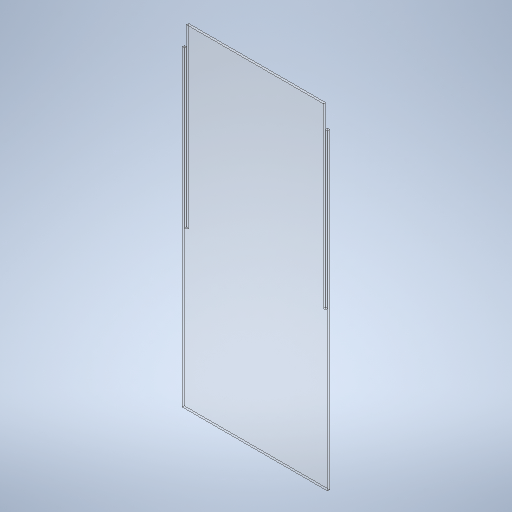
# Autodesk Inventor part: Finishing Sheets .4 ( Front )  Acrylic
Saved by Autodesk Inventor 2025.4 (Build 294407000, 407)
## iProperties
Created: 2026-04-04
Part Number: Finishing Sheets .4 ( Front )  Acrylic
Material: PMMA Plastic
Document SubType Name: Sheet Metal
Designer: lenovo
Density: 1.188 g/cm^3
Sheet Metal Rule: Default_mm
Appearance: Polycarbonate - Clear
Author: lenovo
Autodesk Inventor part; units mm, degrees
ref_plane "YZ Plane" through (0, 0, 0) normal (1, 0, 0) x (0, 1, 0)
ref_plane "XZ Plane" through (0, 0, 0) normal (0, 1, 0) x (-1, 0, 0)
ref_plane "XY Plane" through (0, 0, 0) normal (0, 0, 1) x (1, 0, 0)
sketch "Sketch1" plane through (0, 0, 0) normal (0, 0, 1) x (1, 0, 0)
  line L0 (-102.5, -220) -> (102.5, -220)
  line L1 (102.5, -220) -> (102.5, 220)
  line L2 (102.5, 220) -> (-102.5, 220)
  line L3 (-102.5, 220) -> (-102.5, -220)
  line L4 (-102.5, -220) -> (102.5, 220) construction
  line L5 (102.5, -220) -> (-102.5, 220) construction
  line L6 (-96.5, 220) -> (-99.5, 220)
  line L7 (-99.5, 220) -> (-99.5, 0)
  line L8 (-99.5, 0) -> (-96.5, 0)
  line L9 (-96.5, 0) -> (-96.5, 220)
  line L10 (0, 220) -> (0, 0)
  line L11 (99.5, 220) -> (99.5, 0)
  line L12 (99.5, 0) -> (96.5, 0)
  line L13 (96.5, 0) -> (96.5, 220)
  dimension "d0" = 205
  dimension "d1" = 440
  dimension "d2" = 3
  dimension "d3" = 3
  dimension "d4" = 220
  measures "d0" distance of L1.end L2.end
  measures "d1" distance of L0.end L1.end
  measures "d2" distance between parallel lines of L7 L9
  measures "d3" distance between parallel lines of L3 L7
  measures "d4" distance of L8.end L6.start
sketch "Sketch2" plane through (0, 0, 3) normal (0, 0, 1) x (1, 0, 0)
  line L0 (-96.5, 250) -> (96.5, 250)
  line L1 (96.5, 250) -> (96.5, 220)
  line L2 (96.5, 220) -> (-96.5, 220)
  line L3 (-96.5, 220) -> (-96.5, 250)
  line L4 (-96.5, 250) -> (96.5, 220) construction
  line L5 (96.5, 250) -> (-96.5, 220) construction
  line L6 (-96.5, 220) -> (96.5, 220)
  point P0 (0, 0)
  point P1 (0, 235)
  point P2 (0, 220)
  dimension "d6" = 30
  measures "d6" distance of L0.end L1.end
extrude "Plate1" add sketch "Sketch1" along normal blind 3 contours L3 L2 L7 L8 L9 L13 L12 L11 L1 L0
sheet face with bend "Face2" sketch "Sketch2" thickness 3 toward (0, 0, -1) bend radius 3
bend "Bend1"
equation "\"d5\" = Thickness"
equation "\"d7\" = BendRadius"
equation "\"d8\" = BendReliefWidth"
equation "\"d10\" = MinimumRemnant"
equation "\"d9\" = BendReliefDepth"
equation "\"d11\" = TransitionRadius"
equation "\"BendRadius\" = Thickness"
equation "\"BendReliefWidth\" = Thickness"
equation "\"BendReliefDepth\" = 0.5 * Thickness"
equation "\"CornerReliefSize\" = 4 * Thickness"
equation "\"MinimumRemnant\" = 2 * Thickness"
equation "\"TransitionRadius\" = BendRadius"
equation "\"JacobiRadiusSize\" = BendRadius"
equation "\"GapSize\" = Thickness"
equation "\"Thickness\" = 3"
body "Solid1"
